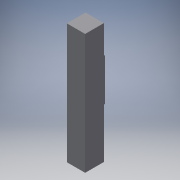
# Autodesk Inventor part: PiezaPuerta-1
Saved by Autodesk Inventor 2017 (Build 210142000, 142)
## iProperties
Created: 2021-02-12
Part Number: PiezaPuerta-1
Material: Generic
Document SubType Name: Modeling
Designer: USUARIO
Density: 1 g/cm^3
Appearance: Default
Author: USUARIO
Autodesk Inventor part; units mm, degrees
ref_plane "YZ Plane" through (0, 0, 0) normal (1, 0, 0) x (0, 1, 0)
ref_plane "XZ Plane" through (0, 0, 0) normal (0, 1, 0) x (-1, 0, 0)
ref_plane "XY Plane" through (0, 0, 0) normal (0, 0, 1) x (1, 0, 0)
sketch "Sketch1" plane through (0, 0, 0) normal (0, 1, 0) x (-1, 0, 0)
  line L0 (0, 0) -> (50.8, 0)
  line L1 (50.8, 0) -> (50.8, -334)
  line L2 (50.8, -334) -> (0, -334)
  line L3 (0, -334) -> (0, 0)
  dimension "d0" = 50.8
  dimension "d1" = 334
  constraints: 8 end point, 2 parallel, 1 horizontal, 1 perpendicular
  measures "d0" distance of L1.end L2.end
  measures "d1" distance of L0.end L1.end
extrude "Extrusion1" add sketch "Sketch1" along normal blind 77.8
sketch "Sketch3" plane through (0, 0, 0) normal (1, 0, 0) x (0, 0, -1)
  line L0 (0, 77.8) -> (121, 77.8)
  line L1 (121, 77.8) -> (121, 52)
  line L2 (121, 52) -> (0, 52)
  line L3 (0, 52) -> (0, 77.8)
  line L4 (0, 77.8) -> (334, 77.8) projected
  line L5 (334, 77.8) -> (217, 77.8)
  line L6 (217, 77.8) -> (217, 52)
  line L7 (217, 52) -> (334, 52)
  line L8 (334, 52) -> (334, 77.8)
  point P0 (0, 0)
  dimension "d9" = 25.8
  dimension "d10" = 117
  dimension "d11" = 25.8
  dimension "d17" = 96
  constraints: 16 end point, 4 parallel, 2 horizontal, 2 perpendicular
  measures "d9" distance of L0.end L1.end
  measures "d10" distance of L7.end L6.end
  measures "d11" distance of L6.end L5.end
  measures "d17" distance between parallel lines of L6 L1
extrude "Extrusion2" cut sketch "Sketch3" against normal blind 50.8
sketch "Sketch6" plane through (0, 77.8, 0) normal (0, 1, 0) x (1, 0, 0)
  line L0 (-50.8, 217) -> (-50.8, 121) projected
  line L1 (0, 217) -> (-50.8, 217) projected
  line L2 (-50.8, 121) -> (-41.8, 121)
  line L3 (-41.8, 121) -> (-41.8, 217)
  line L4 (-41.8, 217) -> (-50.8, 217)
  line L5 (-50.8, 217) -> (-50.8, 121)
  point P0 (0, 0)
  dimension "d18" = 9
  constraints: 8 end point, 2 parallel, 1 horizontal, 1 perpendicular, 1 point on line
  measures "d18" distance of L4.end L3.end
extrude "Extrusion4" cut sketch "Sketch6" against normal blind 25.8
body "Solid1"
